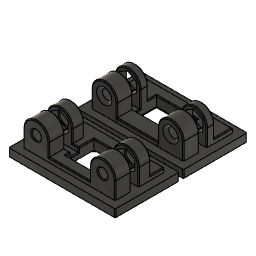
pocket-sdr-panels (Autodesk Fusion 360 design; units mm, degrees)
Autodesk Fusion 360 part; units mm, degrees
sketch "スケッチ1" plane through (0, 0, 0) normal (0, 0, 1) x (1, 0, 0)
  line L0 (0, 0) -> (25, 0)
  line L1 (25, 0) -> (25, 15)
  line L2 (25, 15) -> (0, 15)
  line L3 (0, 15) -> (0, 0)
  line L4 (1.7, 13.3) -> (23.3, 13.3)
  line L5 (23.3, 13.3) -> (23.3, 1.7)
  line L6 (23.3, 1.7) -> (1.7, 1.7)
  line L7 (1.7, 1.7) -> (1.7, 13.3)
  line L8 (-2, 7.2) -> (27, 7.2)
  line L9 (27, 7.2) -> (27, 5.4)
  line L10 (27, 5.4) -> (-2, 5.4)
  line L11 (-2, 5.4) -> (-2, 7.2)
  line L12 (9.2, 10.8) -> (15.8, 10.8)
  line L13 (15.8, 10.8) -> (15.8, 4.2)
  line L14 (15.8, 4.2) -> (9.2, 4.2)
  line L15 (9.2, 4.2) -> (9.2, 10.8)
  circle A0 centre (12.5, 7.5) radius 5
  line L16 (0, 15.9) -> (25, 15.9)
  line L17 (25, 15.9) -> (25, 30.9)
  line L18 (25, 30.9) -> (0, 30.9)
  line L19 (0, 30.9) -> (0, 15.9)
  line L20 (1.7, 23.1) -> (23.3, 23.1)
  line L21 (23.3, 23.1) -> (23.3, 21.3)
  line L22 (23.3, 21.3) -> (1.7, 21.3)
  line L23 (1.7, 21.3) -> (1.7, 23.1)
  line L24 (7.7, 22.2) -> (17.3, 22.2)
  line L25 (17.3, 22.2) -> (17.3, 27)
  line L26 (17.3, 27) -> (7.7, 27)
  line L27 (7.7, 27) -> (7.7, 22.2)
  line L28 (7.4, 21.9) -> (17.6, 21.9)
  line L29 (17.6, 21.9) -> (17.6, 27.3)
  line L30 (17.6, 27.3) -> (7.4, 27.3)
  line L31 (7.4, 27.3) -> (7.4, 21.9)
  dimension "d81" = 10
  dimension "d101" = 21.6
  dimension "d102" = 1.8
  dimension "d235" = 25
  dimension "d236" = 15
  dimension "d239" = 6.6
  dimension "d240" = 6.6
  dimension "d241" = 9.6
  dimension "d242" = 4.8
  dimension "d244" = 11.6
  dimension "d245" = 21.6
  dimension "d270" = 1.8
  dimension "d271" = 5.4
  dimension "d272" = 5.4
  dimension "d273" = 15
  dimension "d274" = 1.7
  dimension "d275" = 1.7
  constraint horizontal L0
  constraint vertical L1
  constraint horizontal L2
  constraint vertical L3
  constraint coincident L0.start L3.end
  constraint horizontal L4
  constraint vertical L5
  constraint horizontal L6
  constraint vertical L7
  constraint horizontal L8
  constraint vertical L9
  constraint horizontal L10
  constraint vertical L11
  constraint horizontal L12
  constraint vertical L13
  constraint horizontal L14
  constraint vertical L15
  constraint horizontal L16
  constraint vertical L17
  constraint horizontal L18
  constraint vertical L19
  constraint horizontal L20
  constraint vertical L21
  constraint horizontal L22
  constraint vertical L23
  constraint horizontal L24
  constraint vertical L25
  constraint horizontal L26
  constraint vertical L27
  constraint horizontal L28
  constraint vertical L29
  constraint horizontal L30
  constraint vertical L31
  measures "d81" diameter of A0
  measures "d101" distance of L20.start L20.end
  measures "d102" distance of L20.start L22.end
  measures "d235" distance of L0.start L0.end
  measures "d236" distance of L0.start L2.end
  measures "d239" distance of L13.end L14.end
  measures "d240" distance of L12.start L14.end
  measures "d241" distance of L24.start L24.end
  measures "d242" distance of L24.start L26.end
  measures "d244" distance of L4.start L6.end
  measures "d245" distance of L5.end L6.end
  measures "d270" distance of L8.start L10.end
  measures "d271" distance of L16 L22
  measures "d272" distance of L0 L10
  measures "d273" distance of L16 L18
  measures "d274" distance of L0 L6
  measures "d275" distance of L3 L7
sketch "スケッチ5" plane through (0, 0, 0) normal (0, 1, 0) x (1, 0, 0)
  line L0 (23.3, 0) -> (17.3, 0)
  line L1 (17.3, 0) -> (17.3, -9)
  line L2 (17.3, -9) -> (23.3, -9)
  line L3 (23.3, -9) -> (23.3, 0)
  line L4 (1.7, 0) -> (7.7, 0)
  line L5 (7.7, 0) -> (7.7, -9)
  line L6 (7.7, -9) -> (1.7, -9)
  line L7 (1.7, -9) -> (1.7, 0)
  circle A0 centre (20.3, -5.9992) radius 3
  circle A1 centre (4.7, -6) radius 3
  circle A2 centre (20.3, -5.9992) radius 1.1
  circle A3 centre (4.7, -6) radius 1.1
  circle A4 centre (4.7, -6) radius 1.25
  circle A5 centre (20.3, -5.9992) radius 1.25
  circle A6 centre (4.7, -6) radius 1.75
  circle A7 centre (20.3, -5.9992) radius 1.75
  line L8 (20.3, -8.3992) -> (22.3785, -7.1992)
  line L9 (22.3785, -7.1992) -> (22.3785, -4.7992)
  line L10 (22.3785, -4.7992) -> (20.3, -3.5992)
  line L11 (20.3, -3.5992) -> (18.2215, -4.7992)
  line L12 (18.2215, -4.7992) -> (18.2215, -7.1992)
  line L13 (18.2215, -7.1992) -> (20.3, -8.3992)
  line L14 (4.7, -8.4) -> (6.7785, -7.2)
  line L15 (6.7785, -7.2) -> (6.7785, -4.8)
  line L16 (6.7785, -4.8) -> (4.7, -3.6)
  line L17 (4.7, -3.6) -> (2.6215, -4.8)
  line L18 (2.6215, -4.8) -> (2.6215, -7.2)
  line L19 (2.6215, -7.2) -> (4.7, -8.4)
  point P0 (20.3, -5.9992)
  point P1 (4.7, -6)
  point P2 (4.7, -6)
  point P3 (20.3, -5.9992)
  point P4 (20.3, -5.9992)
  point P5 (4.7, -6)
  dimension "d21" = 6
  dimension "d22" = 9
  dimension "d23" = 6
  dimension "d24" = 6
  dimension "d25" = 6
  dimension "d26" = 2.2
  dimension "d27" = 2.2
  dimension "d215" = 2.5
  dimension "d216" = 2.5
  dimension "d276" = 6
  dimension "d277" = 5.9992
  dimension "d279" = 3.5
  dimension "d280" = 3.5
  dimension "d281" = 2.4
  dimension "d282" = 2.4
  constraint horizontal L0
  constraint vertical L1
  constraint horizontal L2
  constraint vertical L3
  constraint horizontal L4
  constraint vertical L5
  constraint horizontal L6
  constraint vertical L7
  constraint concentric A0 A2
  constraint concentric A1 A3
  constraint coincident P4 P3
  constraint coincident P5 P2
  constraint concentric A0 A5
  constraint concentric A1 A6
  constraint concentric A0 A7
  measures "d21" distance of L0.start L0.end
  measures "d22" distance of L0.start L2.end
  measures "d23" distance of L4.start L4.end
  measures "d24" diameter of A0
  measures "d25" diameter of A1
  measures "d26" diameter of A2
  measures "d27" diameter of A3
  measures "d215" diameter of A4
  measures "d216" diameter of A5
  measures "d276" distance of L4 P5
  measures "d277" distance of L0 P4
  measures "d279" diameter of A6
  measures "d280" diameter of A7
  measures "d281" distance of L8.start P4
  measures "d282" distance of L14.start P5
extrude "押し出し28" add sketch "スケッチ1" along normal blind 2 contours L0 L1 L3 L5 L6 L7 L10 | L3 L7 L8 L10 | L1 L5 L8 L10 | L1 L2 L3 L4 L5 L7 L8 | L5 L6 L7 L10 A0 | L7 L8 L10 A0 | L5 L8 L10 A0 | L4 L5 L7 L8 A0 | L8 L10 L15 A0 | L10 L13 L14 L15 A0 | L8 L10 L13 A0 | L8 L12 L13 L15 A0 | L8 L10 L13 L15 | L10 L13 L14 L15 | L8 L12 L13 L15 makes body 1
extrude "押し出し29" add sketch "スケッチ1" along normal blind 3 contours L5 L6 L7 L10 A0 | L7 L8 L10 A0 | L5 L8 L10 A0 | L4 L5 L7 L8 A0 | L8 L10 L15 A0 | L10 L13 L14 L15 A0 | L8 L10 L13 A0 | L8 L12 L13 L15 A0 | L8 L10 L13 L15 | L10 L13 L14 L15 | L8 L12 L13 L15 bodies 1
extrude "押し出し30" cut sketch "スケッチ1" along normal blind 5 from surface at 2 contours L3 L8 L10 L11 | L3 L7 L8 L10 | L1 L5 L8 L10 | L1 L8 L9 L10 | L7 L8 L10 A0 | L5 L8 L10 A0 | L8 L10 L15 A0 | L8 L10 L13 A0 | L8 L10 L13 L15 bodies 1
extrude "押し出し31" add sketch "スケッチ5" along normal blind 3.9 from surface at 1.5 contours L0 L1 L3 A0 | A0 | L4 L5 L7 A1 | A1 | A4 | A5 | A6 | A7 | L8 L9 L10 L11 L12 L13 | L14 L15 L16 L17 L18 L19 bodies 1
extrude "押し出し32" add sketch "スケッチ5" along normal blind 1.8 from surface at 7.2 contours L0 L1 L3 A0 | A0 | L4 L5 L7 A1 | A1 bodies 1
copy_body "ボディのコピーと貼り付け1" bodies 1 makes body 2
move_body "移動1" bodies 2 to x (1, 0, 0) y (0, 1, 0) z (0, 0, 1) at (0, 17, 0)
move_body "移動2" bodies 2 to x (1, 0, 0) y (0, 1, 0) z (0, 0, 1) at (0, -1, 0)
extrude "押し出し33" cut sketch "スケッチ1" along normal blind 10 from surface at -1 contours L8 L10 L13 L15 | L10 L13 L14 L15 | L8 L12 L13 L15 bodies 1
extrude "押し出し34" cut sketch "スケッチ1" along normal blind 0.5 contours L8 L10 L15 A0 | L10 L13 L14 L15 A0 | L8 L10 L13 A0 | L8 L12 L13 L15 A0 | L8 L10 L13 L15 | L10 L13 L14 L15 | L8 L12 L13 L15 bodies 1
extrude "押し出し35" cut sketch "スケッチ1" along normal blind 10 from surface at -1 contours L20 L25 L26 L27 | L20 L24 L25 L27 bodies 2
extrude "押し出し36" cut sketch "スケッチ1" along normal blind 0.5 contours L20 L25 L26 L27 L29 L30 L31 | L20 L24 L25 L27 L28 L29 L31 | L20 L25 L26 L27 | L20 L24 L25 L27 bodies 2
chamfer "面取り5" distance 0.2 angle 45 8 edges at (12.5, 10.8, 0.5) (15.8, 7.5, 0.5) (12.5, 4.2, 0.5) (9.2, 7.5, 0.5) (12.5, 27, 0.5) (17.3, 24.6, 0.5) (12.5, 22.2, 0.5) (7.7, 24.6, 0.5) on bodies 1 2
move_body "移動25" bodies 2 to x (1, 0, 0) y (0, 1, 0) z (0, 0, 1) at (0, 24, 0)
sketch "スケッチ12" plane through (0, 0, 0) normal (0, 0, 1) x (1, 0, 0)
  line L0 (0, 15) -> (25, 15)
  line L1 (25, 15) -> (25, 0)
  line L2 (25, 0) -> (0, 0)
  line L3 (0, 0) -> (0, 15)
  line L4 (1.5, 13.5) -> (23.5, 13.5)
  line L5 (23.5, 13.5) -> (23.5, 1.5)
  line L6 (23.5, 1.5) -> (1.5, 1.5)
  line L7 (1.5, 1.5) -> (1.5, 13.5)
  constraint horizontal L0
  constraint vertical L1
  constraint horizontal L2
  constraint vertical L3
  constraint horizontal L4
  constraint vertical L5
  constraint horizontal L6
  constraint vertical L7
move_body "移動26" bodies 2 to x (-1, 0, 0) y (0, 1, 0) z (0, 0, -1) at (23, -38, 57)
move_body "移動27" bodies 2 to x (1, 0, 0) y (0, 1, 0) z (0, 0, 1) at (2, -2, 2)
chamfer "面取り17" distance 0.9 angle 45 2 edges at (21.3256, 1.5, 53.3978) (5.7256, 1.5, 53.3986) on bodies 2
extrude "押し出し67" cut sketch "スケッチ1" along normal blind 10 from surface at 2 contours L0 L1 L3 L5 L6 L7 L10 | L3 L7 L8 L10 | L1 L5 L8 L10 | L1 L2 L3 L4 L5 L7 L8 bodies 1
extrude "押し出し68" cut sketch "スケッチ1" against normal blind 10 from surface at 57 contours L0 L1 L3 L5 L6 L7 L10 | L3 L7 L8 L10 | L1 L5 L8 L10 | L1 L2 L3 L4 L5 L7 L8 bodies 2
chamfer "面取り26" distance 0.2 angle 45 2 edges at (3.6744, 1.7, 5.6022) (19.2744, 1.7, 5.6014) on bodies 1
chamfer "面取り28" distance 0.2 angle 45 2 edges at (19.2744, 5.4, 5.6014) (3.6744, 5.4, 5.6022) on bodies 1
chamfer "面取り29" distance 0.2 angle 45 12 edges at (25, 7.5, 59) (12.5, 0, 59) (12.5, 15, 59) (0, 7.5, 59) (0, 0, 58) (0, 15, 58) (25, 15, 58) (25, 0, 58) (17.6, 8.6, 59) (12.5, 11.3, 59) (7.4, 8.6, 59) (12.5, 5.9, 59) on bodies 2
move_body "移動47" bodies 2 to x (-1, 0, 0) y (0, 1, 0) z (0, 0, -1) at (51, 0, 59)
move_body "Move60" bodies 2 to x (1, 0, 0) y (0, 1, 0) z (0, 0, 1) at (-26, 16, 0)
extrude "Extrude72" add sketch "スケッチ5" along normal blind 1 from surface at 9 contours L0 L1 L3 A0 | A0 | L4 L5 L7 A1 | A1 | L8 L9 L10 L11 L12 L13 | L14 L15 L16 L17 L18 L19 bodies 1
chamfer "Chamfer35" distance 0.2 angle 45 7 edges at (4.6999, 1.7, 9) (7.7, 1.7, 4.5001) (1.7, 1.7, 4) (12.5, 1.7, 3) (17.3, 1.7, 4.4996) (20.3, 1.7, 8.9992) (23.3, 1.7, 3.9996) on bodies 1
chamfer "Chamfer36" distance 0.2 angle 45 1 edges at (12.5, 17.7, 3) on bodies 2
chamfer "Chamfer37" distance 0.2 angle 45 6 edges at (7.7, 17.7, 4.4001) (1.7, 17.7, 4) (4.6998, 17.7, 9) (17.3, 17.7, 4.3996) (20.3, 17.7, 8.9992) (23.3, 17.7, 3.9996) on bodies 2
chamfer "Chamfer40" distance 0.2 angle 45 7 edges at (23.3, 21.4, 3.9996) (20.3, 21.4, 8.9992) (17.3, 21.4, 4.4996) (12.5, 21.4, 3) (7.7, 21.4, 4.5001) (1.7, 21.4, 4) (4.6998, 21.4, 9) on bodies 2
chamfer "Chamfer41" distance 0.2 angle 45 10 edges at (23.3, 5.4, 3.9996) (20.3, 5.4, 8.9992) (17.3, 5.4, 4.4996) (16.55, 5.4, 3) (15.8, 5.4, 2.5) (9.2, 5.4, 2.5) (8.45, 5.4, 3) (7.7, 5.4, 4.5001) (1.7, 5.4, 4) (4.6999, 5.4, 9) on bodies 1
chamfer "Chamfer42" distance 0.2 angle 45 10 edges at (1.7, 7.2, 4) (4.6999, 7.2, 9) (7.7, 7.2, 4.5001) (8.45, 7.2, 3) (9.2, 7.2, 2.5) (15.8, 7.2, 2.5) (16.55, 7.2, 3) (17.3, 7.2, 4.4996) (20.3, 7.2, 8.9992) (23.3, 7.2, 3.9996) on bodies 1
chamfer "Chamfer46" distance 0.2 angle 45 8 edges at (15.8, 9.1, 3) (15.8, 6.3, 2) (15.8, 4.7, 3) (12.5, 4.2, 3) (9.2, 4.7, 3) (9.2, 6.3, 2) (9.2, 9.1, 3) (12.5, 10.8, 3) on bodies 1
chamfer "Chamfer47" distance 0.2 angle 45 12 edges at (12.5, 29.3, 3) (23.3, 27.15, 3) (23.3, 25, 4.4996) (17.3, 25, 4.4996) (20.3, 25, 8.9992) (17.3, 26, 3) (12.5, 27, 3) (7.7, 26, 3) (7.7, 25, 4.5001) (1.7, 25, 4.5) (4.6998, 25, 9) (1.7, 27.15, 3) on bodies 2
chamfer "Chamfer48" distance 0.2 angle 45 9 edges at (1.7, 23.2, 4) (4.6998, 23.2, 9) (7.7, 23.2, 4.0001) (7.7, 22.7, 2) (12.5, 22.2, 2) (17.3, 22.7, 2) (17.3, 23.2, 3.9996) (23.3, 23.2, 3.9996) (20.3, 23.2, 8.9992) on bodies 2
chamfer "Chamfer49" distance 0.2 angle 45 11 edges at (23.3, 10, 4.4996) (17.3, 10, 4.4996) (20.3, 10, 8.9992) (7.7, 10, 4.5001) (1.7, 10, 4.5) (4.6999, 10, 9) (1.7, 11.65, 3) (1.7, 13.3, 2.5) (12.5, 13.3, 3) (23.3, 11.65, 3) (23.3, 13.3, 2.5) on bodies 1
chamfer "Chamfer50" distance 0.2 angle 45 1 edges at (7.8384, 5.6919, 0) on bodies 1
chamfer "Chamfer51" distance 0.2 angle 45 8 edges at (12.5, 0, 0) (0, 7.5, 0) (12.5, 15, 0) (25, 7.5, 0) (0, 0, 1) (25, 0, 1) (0, 15, 1) (25, 15, 1) on bodies 1
chamfer "Chamfer52" distance 0.2 angle 45 6 edges at (22.3785, 24.1, 4.7992) (20.3, 24.1, 3.5992) (18.2215, 24.1, 4.7992) (18.2215, 24.1, 7.1992) (20.3, 24.1, 8.3992) (22.3785, 24.1, 7.1992) on bodies 2
chamfer "Chamfer53" distance 0.2 angle 45 6 edges at (6.7785, 24.1, 7.2) (4.7, 24.1, 8.4) (6.7785, 24.1, 4.8) (4.7, 24.1, 3.6) (2.6215, 24.1, 7.2) (2.6215, 24.1, 4.8) on bodies 2
chamfer "Chamfer54" distance 0.2 angle 45 6 edges at (18.2215, 8.1, 4.7992) (20.3, 8.1, 3.5992) (22.3785, 8.1, 4.7992) (22.3785, 8.1, 7.1992) (20.3, 8.1, 8.3992) (18.2215, 8.1, 7.1992) on bodies 1
chamfer "Chamfer55" distance 0.2 angle 45 6 edges at (6.7785, 8.1, 7.2) (6.7785, 8.1, 4.8) (2.6215, 8.1, 4.8) (4.7, 8.1, 3.6) (2.6215, 8.1, 7.2) (4.7, 8.1, 8.4) on bodies 1
named bodies: "FRONT", "BACK"
